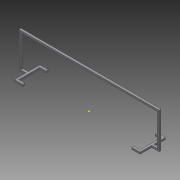
# Autodesk Inventor part: CameraMount
Saved by Autodesk Inventor 2015 (Build 190159000, 159)
## iProperties
Created: 2016-12-16
Part Number: CameraMount
Material: Generic
Document SubType Name: Modeling
Designer: Guy
Density: 1 g/cm^3
Appearance: Default
Author: Guy
Autodesk Inventor part; units mm, degrees
ref_plane "YZ Plane" through (0, 0, 0) normal (1, 0, 0) x (0, 1, 0)
ref_plane "XZ Plane" through (0, 0, 0) normal (0, 1, 0) x (-1, 0, 0)
ref_plane "XY Plane" through (0, 0, 0) normal (0, 0, 1) x (1, 0, 0)
sketch "Sketch1" plane through (0, 0, 0) normal (0, 0, 1) x (1, 0, 0)
  line L0 (0, 0) -> (-1440, 0)
  line L1 (-1440, 0) -> (-1440, 20)
  line L2 (-1440, 20) -> (0, 20)
  line L3 (0, 20) -> (0, 0)
  dimension "d0" = 1440
  dimension "d1" = 20
  constraints: 8 end point, 2 parallel, 1 horizontal, 1 perpendicular
  measures "d0" distance of L1.end L2.end
  measures "d1" distance of L2.end L0.start
extrude "Extrusion1" add sketch "Sketch1" along normal blind 20
sketch "Sketch2" plane through (0, 0, 20) normal (0, 0, 1) x (1, 0, 0)
  line L0 (-1440, 0) -> (0, 0) projected
  line L1 (0, 0) -> (0, 20) projected
  line L2 (0, 20) -> (-1440, 20) projected
  line L3 (-1440, 20) -> (-1440, 0) projected
  line L4 (0, 0) -> (-20, 0)
  line L5 (-20, 0) -> (-20, 20)
  line L6 (-20, 20) -> (0, 20)
  line L7 (0, 20) -> (0, 0)
  line L8 (-1440, 0) -> (-1420, 0)
  line L9 (-1420, 0) -> (-1420, 20)
  line L10 (-1420, 20) -> (-1440, 20)
  line L11 (-1440, 20) -> (-1440, 0)
  dimension "d4" = 20
  dimension "d5" = 20
  constraints: 16 end point, 4 parallel, 2 horizontal, 2 perpendicular, 2 point on line
  measures "d4" distance between parallel lines of L1 L5
  measures "d5" distance between parallel lines of L3 L9
extrude "Extrusion2" add sketch "Sketch2" along normal blind 350 contours L3 L2 L9 L0 | L5 L2 L1 L0
ref_plane "Work Plane1" through (-720, 0, 0) normal (1, 0, 0) x (0, 0, -1)
sketch "Sketch3" plane through (-720, 0, 0) normal (1, 0, 0) x (0, 0, -1)
  point P0 (0, 0)
sketch "Sketch4" plane through (-720, 0, 0) normal (1, 0, 0) x (0, 0, -1)
  line L0 (-20, 20) -> (-20, 0) projected
  line L1 (0, 0) -> (0, 20) projected
  line L2 (0, 0) -> (-370, 0) projected
  line L3 (-370, 20) -> (-370, 0) projected
  line L4 (0, 20) -> (-370, 20) projected
  line L5 (-20, 20) -> (0, 20)
  line L6 (0, 20) -> (0, 0)
  line L7 (0, 0) -> (-20, 0)
  line L8 (-20, 0) -> (-20, 20)
  point P0 (0, 0)
  constraints: 8 end point, 2 parallel, 1 horizontal, 1 perpendicular
extrude "Extrusion3" cut sketch "Sketch4" along normal mid plane 1250 contours L4 L1 L2 L0
sketch "Sketch5" plane through (-1420, 0, 20) normal (1, 0, 0) x (0, 0, -1)
  line L0 (0, 20) -> (0, 0) projected
  line L1 (0, 20) -> (-350, 20) projected
  line L2 (-350, 0) -> (-350, 20) projected
  line L3 (0, 0) -> (-350, 0) projected
  line L4 (-350, 0) -> (-330, 0)
  line L5 (-330, 0) -> (-330, 20)
  line L6 (-330, 20) -> (-350, 20)
  line L7 (-350, 20) -> (-350, 0)
  point P0 (20, 0)
  dimension "d14" = 20
  constraints: 8 end point, 2 parallel, 1 horizontal, 1 perpendicular, 1 point on line
  measures "d14" distance between parallel lines of L2 L5
extrude "Extrusion4" add sketch "Sketch5" along normal blind 1401 contours L5 L3 L2 L1
sketch "Sketch7" plane through (-1440, 0, 370) normal (0, -1, 0) x (1, 0, 0)
  line L0 (95, -370) -> (95, -350) projected
  line L1 (20, -350) -> (95, -350) projected
  line L2 (20, -350) -> (20, -20) projected
  line L3 (20, -20) -> (1420, -20) projected
  line L4 (1420, -350) -> (1420, -20) projected
  line L5 (1345, -350) -> (1420, -350) projected
  line L6 (1345, -350) -> (1345, -370) projected
  line L7 (1440, -370) -> (1345, -370) projected
  line L8 (1440, -370) -> (1440, 0) projected
  line L9 (0, 0) -> (1440, 0) projected
  line L10 (0, -370) -> (0, 0) projected
  line L11 (95, -370) -> (0, -370) projected
  line L12 (1345, -370) -> (1365, -370)
  line L13 (1365, -370) -> (1365, -350)
  line L14 (1365, -350) -> (1345, -350)
  line L15 (1345, -350) -> (1345, -370)
  line L16 (20, -350) -> (95, -350) projected
  line L17 (95, -370) -> (75, -370)
  line L18 (75, -370) -> (75, -350)
  line L19 (75, -350) -> (95, -350)
  line L20 (95, -350) -> (95, -370)
  dimension "d23" = 20
  dimension "d24" = 20
  constraints: 16 end point, 4 parallel, 2 horizontal, 2 perpendicular, 2 point on line
  measures "d23" distance between parallel lines of L6 L13
  measures "d24" distance between parallel lines of L18 L0
extrude "Extrusion6" add sketch "Sketch7" along normal blind 120 contours L11 L18 L1 L0 | L7 L6 L5 L13
sketch "Sketch8" plane through (-1440, 20, 370) normal (0, 1, 0) x (1, 0, 0)
  line L0 (95, 350) -> (95, 370) projected
  line L1 (0, 370) -> (95, 370) projected
  line L2 (0, 370) -> (0, 0) projected
  line L3 (1440, 0) -> (0, 0) projected
  line L4 (1440, 370) -> (1440, 0) projected
  line L5 (1345, 370) -> (1440, 370) projected
  line L6 (1345, 370) -> (1345, 350) projected
  line L7 (1420, 350) -> (1345, 350) projected
  line L8 (1420, 350) -> (1420, 20) projected
  line L9 (20, 20) -> (1420, 20) projected
  line L10 (20, 350) -> (20, 20) projected
  line L11 (95, 350) -> (20, 350) projected
  line L12 (1345, 370) -> (1365, 370)
  line L13 (1365, 370) -> (1365, 350)
  line L14 (1365, 350) -> (1345, 350)
  line L15 (1345, 350) -> (1345, 370)
  line L16 (95, 370) -> (75, 370)
  line L17 (75, 370) -> (75, 350)
  line L18 (75, 350) -> (95, 350)
  line L19 (95, 350) -> (95, 370)
  dimension "d27" = 20
  dimension "d28" = 20
  constraints: 16 end point, 4 parallel, 2 horizontal, 2 perpendicular, 2 point on line
  measures "d27" distance between parallel lines of L6 L13
  measures "d28" distance between parallel lines of L0 L17
extrude "Extrusion7" add sketch "Sketch8" along normal blind 120 contours L11 L17 L1 L0 | L7 L6 L5 L13
sketch "Sketch9" plane through (-1345, 0, 0) normal (1, 0, 0) x (0, 0, -1)
  line L0 (-20, -120) -> (-20, 140) projected
  line L1 (0, -120) -> (-20, -120) projected
  line L2 (0, 140) -> (0, -120) projected
  line L3 (-20, 140) -> (0, 140) projected
  line L4 (-20, -120) -> (0, -120)
  line L5 (0, -120) -> (0, -100)
  line L6 (0, -100) -> (-20, -100)
  line L7 (-20, -100) -> (-20, -120)
  line L8 (0, 140) -> (0, -120) projected
  line L9 (-20, 140) -> (0, 140)
  line L10 (0, 140) -> (0, 120)
  line L11 (0, 120) -> (-20, 120)
  line L12 (-20, 120) -> (-20, 140)
  point P0 (0, 0)
  dimension "d35" = 20
  dimension "d36" = 20
  constraints: 16 end point, 4 parallel, 2 horizontal, 2 perpendicular, 2 point on line
  measures "d35" distance between parallel lines of L3 L11
  measures "d36" distance between parallel lines of L1 L6
extrude "Extrusion8" add sketch "Sketch9" along normal blind 1251 contours L0 L6 L2 L1 | L0 L3 L2 L11
sketch "Sketch10" plane through (-720, 0, 0) normal (1, 0, 0) x (0, 0, -1)
  line L0 (0, 0) -> (-20, 0) projected
  line L1 (0, 0) -> (0, -120) projected
  line L2 (-20, -120) -> (0, -120) projected
  line L3 (-20, 0) -> (-20, -120) projected
  line L4 (0, 120) -> (-20, 120) projected
  line L5 (0, 140) -> (-20, 140) projected
  line L6 (-20, 20) -> (-20, 140) projected
  line L7 (0, 20) -> (0, 140) projected
  line L8 (-20, -100) -> (0, -100) projected
  line L9 (-20, -120) -> (0, -120)
  line L10 (0, -120) -> (0, -100)
  line L11 (0, -100) -> (-20, -100)
  line L12 (-20, -100) -> (-20, -120)
  line L13 (-20, 120) -> (0, 120)
  line L14 (0, 120) -> (0, 140)
  line L15 (0, 140) -> (-20, 140)
  line L16 (-20, 140) -> (-20, 120)
  point P0 (0, 0)
  constraints: 16 end point, 4 parallel, 2 horizontal, 2 perpendicular
extrude "Extrusion9" cut sketch "Sketch10" along normal mid plane 1120.8 contours L1 L2 L3 L8 | L4 L6 L5 L7
body "Solid1"
